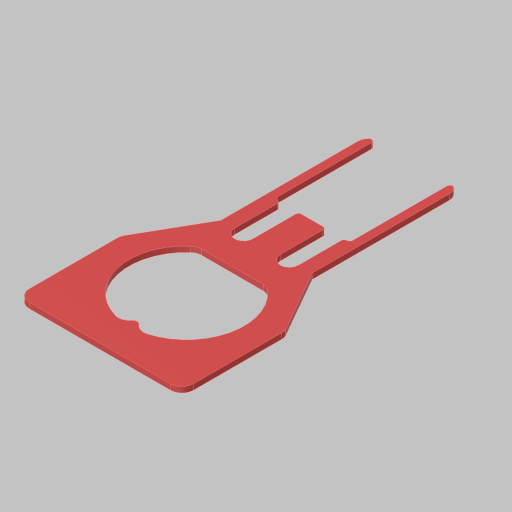
# Autodesk Inventor part: EL2-037
Saved by Autodesk Inventor 2023.5 (Build 275446000, 446)
## iProperties
Created: 2025-01-21
Part Number: EL2-037
Material: ABS Plastic
Document SubType Name: Modeling
Designer: slick
Density: 1.06 g/cm^3
Appearance: Smooth - Red
Author: slick
Autodesk Inventor part; units mm, degrees
ref_plane "YZ Plane" through (0, 0, 0) normal (1, 0, 0) x (0, 1, 0)
ref_plane "XZ Plane" through (0, 0, 0) normal (0, 1, 0) x (-1, 0, 0)
ref_plane "XY Plane" through (0, 0, 0) normal (0, 0, 1) x (1, 0, 0)
sketch "Sketch1" plane through (0, 0, 0) normal (0, 1, 0) x (-1, 0, 0)
  line L0 (8.89, 0) -> (-8.89, 0) construction
  line L1 (8.89, 1.5875) -> (-8.89, 1.5875)
  line L2 (-8.89, -1.5875) -> (8.89, -1.5875)
  arc A0 (8.89, -1.5875) -> (8.89, 1.5875) centre (8.89, 0) ccw
  arc A1 (-8.89, 1.5875) -> (-8.89, -1.5875) centre (-8.89, 0) ccw
  line L3 (8.89, -5.0038) -> (-8.89, -5.0038) construction
  line L4 (8.89, -3.4163) -> (-8.89, -3.4163)
  line L5 (-8.89, -6.5913) -> (8.89, -6.5913)
  arc A2 (8.89, -6.5913) -> (8.89, -3.4163) centre (8.89, -5.0038) ccw
  arc A3 (-8.89, -3.4163) -> (-8.89, -6.5913) centre (-8.89, -5.0038) ccw
  line L6 (8.89, -10.0076) -> (-8.89, -10.0076) construction
  line L7 (8.89, -8.4201) -> (-8.89, -8.4201)
  line L8 (-8.89, -11.5951) -> (8.89, -11.5951)
  arc A4 (8.89, -11.5951) -> (8.89, -8.4201) centre (8.89, -10.0076) ccw
  arc A5 (-8.89, -8.4201) -> (-8.89, -11.5951) centre (-8.89, -10.0076) ccw
  line L9 (12.7, 32.8549) -> (-12.7, 32.8549)
  line L10 (-12.7, 32.8549) -> (-12.7, -17.9451)
  line L11 (-12.7, -17.9451) -> (12.7, -17.9451)
  line L12 (12.7, -17.9451) -> (12.7, 32.8549)
  line L13 (6.35, 26.5049) -> (-6.35, 26.5049) construction
  arc A6 (8.89, -16.5989) -> (8.89, -13.4239) centre (8.89, -15.0114) ccw
  line L14 (-8.89, -16.5989) -> (8.89, -16.5989)
  arc A7 (-8.89, -13.4239) -> (-8.89, -16.5989) centre (-8.89, -15.0114) ccw
  line L15 (8.89, -13.4239) -> (-8.89, -13.4239)
  point P0 (0, 0)
  point P1 (0, -5.0038)
  point P2 (0, -10.0076)
  point P3 (10.4775, -5.0038)
  point P4 (10.4775, 0)
  point P5 (10.4775, -10.0076)
  point P6 (0, -17.9451)
  point P7 (0, -11.5951)
  point P8 (0, 26.5049)
  point P9 (0, 32.8549)
  point P10 (10.4775, -15.0114)
  point P11 (0, -16.5989)
  dimension "d1" = 17.78
  dimension "d3" = 3.175
  dimension "d4" = 5.0038
  dimension "d5" = 5.0038
  dimension "d8" = 25.4
  dimension "d9" = 50.8
  dimension "d10" = 6.35
  dimension "d11" = 12.7
  dimension "d12" = 6.35
  dimension "d43" = 5.0038
  constraints: 38 end point, 19 point on circle, 12 tangent, 9 parallel, 8 centre point, 7 midpoint, 4 vertical alignment, 3 horizontal, 2 equal radius, 1 horizontal alignment, 1 perpendicular, 1 vertical, 12 other
  measures "d1" distance of L1.start L1.end
  measures "d3" distance between parallel lines of L2 L1
  measures "d4" distance of point (10.477, -5.004) point (10.477, 0)
  measures "d5" distance of point (10.477, -10.008) point (10.477, -5.004)
  measures "d8" distance of L10.end L11.end
  measures "d9" distance of L11.end L9.start
  measures "d10" distance of point (0, -11.595) point (0, -17.945)
  measures "d11" distance of L13.start L13.end
  measures "d12" distance from line of L9 L13.start
  measures "d43" distance of L6.start A6.centre
extrude "Extrusion1" add sketch "Sketch1" along normal blind 6.35 contours A0 L2 A1 L1 | A2 L5 A3 L4 | A4 L8 A5 L7 | L12 L11 L10 L9 | L14 A7 L15 A6
fillet "Fillet1" radius 3.175 4 edges at (-12.7, 3.175, -17.9451) (12.7, 3.175, -17.9451) (12.7, 3.175, 32.8549) (-12.7, 3.175, 32.8549)
sketch "Sketch2" plane through (0, 6.35, 0) normal (0, 1, 0) x (1, 0, 0)
  line L0 (-6.35, -10.6299) -> (-6.35, -23.3299) construction
  line L1 (-8.9027, -10.6299) -> (-8.9027, -23.3299)
  line L2 (-3.7973, -23.3299) -> (-3.7973, -10.6299)
  arc A0 (-3.7973, -10.6299) -> (-8.9027, -10.6299) centre (-6.35, -10.6299) ccw
  arc A1 (-8.9027, -23.3299) -> (-3.7973, -23.3299) centre (-6.35, -23.3299) ccw
  line L3 (6.35, -10.6299) -> (6.35, -23.3299) construction
  line L4 (3.7973, -10.6299) -> (3.7973, -23.3299)
  line L5 (8.9027, -23.3299) -> (8.9027, -10.6299)
  arc A2 (8.9027, -10.6299) -> (3.7973, -10.6299) centre (6.35, -10.6299) ccw
  arc A3 (3.7973, -23.3299) -> (8.9027, -23.3299) centre (6.35, -23.3299) ccw
  line L6 (-9.525, -32.8549) -> (9.525, -32.8549) projected
  line L7 (9.525, 17.9451) -> (-9.525, 17.9451) projected
  line L8 (-6.35, -16.9799) -> (6.35, -16.9799) construction
  point P0 (0, 0)
  point P1 (0, -16.9799)
  point P2 (0, 17.9451)
  dimension "d23" = 5.1054
  dimension "d24" = 12.7
  dimension "d26" = 34.925
  dimension "d27" = 12.7
  constraints: 18 end point, 8 point on circle, 8 tangent, 4 centre point, 4 midpoint, 3 parallel, 2 horizontal alignment, 1 equal radius, 1 perpendicular, 1 vertical, 1 vertical alignment
  measures "d23" diameter of A1
  measures "d24" distance of L0.start L0.end
  measures "d26" distance from line of L8.start L7
  measures "d27" distance of L8.start L8.end
extrude "Extrusion2" cut sketch "Sketch2" against normal blind 25.4
sketch "Sketch3" plane through (0, 6.35, 0) normal (0, 1, 0) x (1, 0, 0)
  circle A0 centre (0, -45.5549) radius 16.002
  line L0 (-9.525, -32.8549) -> (9.525, -32.8549) projected
  circle A1 centre (0, -45.5549) radius 19.177
  line L1 (3.7973, -10.6299) -> (3.7973, -23.3299) projected
  arc A2 (3.7973, -23.3299) -> (8.9027, -23.3299) centre (6.35, -23.3299) ccw projected
  line L2 (8.9027, -23.3299) -> (8.9027, -10.6299) projected
  arc A3 (8.9027, -10.6299) -> (3.7973, -10.6299) centre (6.35, -10.6299) ccw projected
  line L3 (-8.9027, -10.6299) -> (-8.9027, -23.3299) projected
  arc A4 (-8.9027, -23.3299) -> (-3.7973, -23.3299) centre (-6.35, -23.3299) ccw projected
  line L4 (-3.7973, -23.3299) -> (-3.7973, -10.6299) projected
  arc A5 (-3.7973, -10.6299) -> (-8.9027, -10.6299) centre (-6.35, -10.6299) ccw projected
  arc A6 (-12.7, -29.6799) -> (-9.525, -32.8549) centre (-9.525, -29.6799) ccw projected
  line L5 (-12.7, -29.6799) -> (-12.7, 14.7701) projected
  arc A7 (-9.525, 17.9451) -> (-12.7, 14.7701) centre (-9.525, 14.7701) ccw projected
  line L6 (-9.525, 17.9451) -> (9.525, 17.9451) projected
  arc A8 (12.7, 14.7701) -> (9.525, 17.9451) centre (9.525, 14.7701) ccw projected
  line L7 (12.7, 14.7701) -> (12.7, -29.6799) projected
  arc A9 (9.525, -32.8549) -> (12.7, -29.6799) centre (9.525, -29.6799) ccw projected
  line L8 (9.525, -32.8549) -> (-9.525, -32.8549) projected
  line L9 (3.7973, -10.6299) -> (3.7973, -23.3299) projected
  arc A10 (3.7973, -23.3299) -> (8.9027, -23.3299) centre (6.35, -23.3299) ccw projected
  line L10 (8.9027, -23.3299) -> (8.9027, -10.6299) projected
  arc A11 (8.9027, -10.6299) -> (3.7973, -10.6299) centre (6.35, -10.6299) ccw projected
  line L11 (-8.9027, -10.6299) -> (-8.9027, -23.3299) projected
  arc A12 (-8.9027, -23.3299) -> (-3.7973, -23.3299) centre (-6.35, -23.3299) ccw projected
  line L12 (-3.7973, -23.3299) -> (-3.7973, -10.6299) projected
  arc A13 (-3.7973, -10.6299) -> (-8.9027, -10.6299) centre (-6.35, -10.6299) ccw projected
  arc A14 (-12.7, -29.6799) -> (-9.525, -32.8549) centre (-9.525, -29.6799) ccw projected
  line L13 (-12.7, -29.6799) -> (-12.7, 14.7701) projected
  arc A15 (-9.525, 17.9451) -> (-12.7, 14.7701) centre (-9.525, 14.7701) ccw projected
  line L14 (-9.525, 17.9451) -> (9.525, 17.9451) projected
  arc A16 (12.7, 14.7701) -> (9.525, 17.9451) centre (9.525, 14.7701) ccw projected
  line L15 (12.7, 14.7701) -> (12.7, -29.6799) projected
  arc A17 (9.525, -32.8549) -> (12.7, -29.6799) centre (9.525, -29.6799) ccw projected
  line L16 (9.525, -32.8549) -> (-9.525, -32.8549) projected
  point P0 (0, 0)
  point P1 (0, -32.8549)
  point P2 (12.433012, -30.954299)
  point P3 (9.726813, -32.84848)
  point P4 (-9.726813, -32.84848)
  point P5 (-12.433012, -30.954299)
  dimension "d30" = 32.004
  dimension "d31" = 12.7
  dimension "d32" = 3.175
  constraints: 2 centre point, 1 midpoint, 1 vertical alignment
  measures "d30" diameter of A0
  measures "d31" distance from line of L0 A0.centre
  measures "d32" radial gap between concentric circles of A0 A1
extrude "Extrusion3" add sketch "Sketch3" against normal up to surface (6.35 mm away) contours A0 A9 A1 A6 picked at (17.941917, -47.047698)
fillet "Fillet2" radius 3.175 4 edges at (-12.433, 3.175, 30.9543) (12.433, 3.175, 30.9543) (9.7268, 3.175, 32.8485) (-9.7268, 3.175, 32.8485)
sketch "Sketch4" plane through (0, 6.35, 0) normal (0, 1, 0) x (1, 0, 0)
  circle A0 centre (0, -60.4901) radius 1.1811
  arc A1 (-8.59106, -32.8549) -> (-10.717559, -33.672227) centre (-8.59106, -36.0299) ccw
  arc A2 (-10.717559, -33.672227) -> (10.717559, -33.672227) centre (0, -45.5549) ccw
  arc A3 (10.717559, -33.672227) -> (8.59106, -32.8549) centre (8.59106, -36.0299) ccw
  line L0 (8.59106, -32.8549) -> (-8.59106, -32.8549)
  arc A4 (12.699247, -29.749044) -> (13.618736, -32.053517) centre (15.873494, -29.818188) ccw
  arc A5 (-13.618736, -32.053517) -> (13.618736, -32.053517) centre (0, -45.5549) ccw
  arc A6 (-13.618736, -32.053517) -> (-12.699247, -29.749044) centre (-15.873494, -29.818188) ccw
  arc A7 (-12.7, -29.6799) -> (-12.699247, -29.749044) centre (-9.525, -29.6799) ccw
  line L1 (-12.7, -29.6799) -> (-12.7, 14.7701)
  arc A8 (-9.525, 17.9451) -> (-12.7, 14.7701) centre (-9.525, 14.7701) ccw
  line L2 (-9.525, 17.9451) -> (9.525, 17.9451)
  arc A9 (12.7, 14.7701) -> (9.525, 17.9451) centre (9.525, 14.7701) ccw
  line L3 (12.7, 14.7701) -> (12.7, -29.6799)
  arc A10 (12.699247, -29.749044) -> (12.7, -29.6799) centre (9.525, -29.6799) ccw
  line L4 (3.7973, -10.6299) -> (3.7973, -23.3299)
  arc A11 (3.7973, -23.3299) -> (8.9027, -23.3299) centre (6.35, -23.3299) ccw
  line L5 (8.9027, -23.3299) -> (8.9027, -10.6299)
  arc A12 (8.9027, -10.6299) -> (3.7973, -10.6299) centre (6.35, -10.6299) ccw
  line L6 (-8.9027, -10.6299) -> (-8.9027, -23.3299)
  arc A13 (-8.9027, -23.3299) -> (-3.7973, -23.3299) centre (-6.35, -23.3299) ccw
  line L7 (-3.7973, -23.3299) -> (-3.7973, -10.6299)
  arc A14 (-3.7973, -10.6299) -> (-8.9027, -10.6299) centre (-6.35, -10.6299) ccw
  point P0 (0, 0)
  point P1 (0, -61.5569)
  point P2 (-0.524608, -61.548298)
  point P3 (0.524608, -61.548298)
  dimension "d36" = 2.3622
  dimension "d37" = 1.0668
  constraints: 1 centre point, 1 point on circle
  measures "d36" diameter of A0
  measures "d37" distance of point (0, -61.557) A0.centre
extrude "Extrusion4" add sketch "Sketch4" against normal up to surface (6.35 mm away) contours A0 A2 picked at (-0.032567, -60.808312)
fillet "Fillet3" radius 3.175 2 edges at (0.5246, 3.175, 61.5483) (-0.5246, 3.175, 61.5483)
sketch "Sketch5" plane through (0, 6.35, 0) normal (0, 1, 0) x (1, 0, 0)
  arc A0 (-8.59106, -32.8549) -> (-10.717559, -33.672227) centre (-8.59106, -36.0299) ccw construction
  arc A1 (-10.717559, -33.672227) -> (-4.36514, -60.950015) centre (0, -45.5549) ccw construction
  arc A2 (-4.36514, -60.950015) -> (-0.94872, -59.786588) centre (-3.499041, -57.895428) ccw construction
  arc A3 (0.94872, -59.786588) -> (-0.94872, -59.786588) centre (0, -60.4901) ccw construction
  arc A4 (0.94872, -59.786588) -> (4.36514, -60.950015) centre (3.499041, -57.895428) ccw construction
  arc A5 (4.36514, -60.950015) -> (10.717559, -33.672227) centre (0, -45.5549) ccw construction
  arc A6 (10.717559, -33.672227) -> (8.59106, -32.8549) centre (8.59106, -36.0299) ccw construction
  line L0 (8.59106, -32.8549) -> (-8.59106, -32.8549) construction
  arc A7 (12.699247, -29.749044) -> (13.618736, -32.053517) centre (15.873494, -29.818188) ccw construction
  arc A8 (-13.618736, -32.053517) -> (13.618736, -32.053517) centre (0, -45.5549) ccw construction
  arc A9 (-13.618736, -32.053517) -> (-12.699247, -29.749044) centre (-15.873494, -29.818188) ccw construction
  arc A10 (-12.7, -29.6799) -> (-12.699247, -29.749044) centre (-9.525, -29.6799) ccw construction
  line L1 (-12.7, -29.6799) -> (-12.7, 14.7701) construction
  arc A11 (-9.525, 17.9451) -> (-12.7, 14.7701) centre (-9.525, 14.7701) ccw construction
  line L2 (-9.525, 17.9451) -> (9.525, 17.9451) construction
  arc A12 (12.7, 14.7701) -> (9.525, 17.9451) centre (9.525, 14.7701) ccw construction
  line L3 (12.7, 14.7701) -> (12.7, -29.6799) construction
  arc A13 (12.699247, -29.749044) -> (12.7, -29.6799) centre (9.525, -29.6799) ccw construction
  line L4 (3.7973, -10.6299) -> (3.7973, -23.3299) construction
  arc A14 (3.7973, -23.3299) -> (8.9027, -23.3299) centre (6.35, -23.3299) ccw construction
  line L5 (8.9027, -23.3299) -> (8.9027, -10.6299) construction
  arc A15 (8.9027, -10.6299) -> (3.7973, -10.6299) centre (6.35, -10.6299) ccw construction
  line L6 (-8.9027, -10.6299) -> (-8.9027, -23.3299) construction
  arc A16 (-8.9027, -23.3299) -> (-3.7973, -23.3299) centre (-6.35, -23.3299) ccw construction
  line L7 (-3.7973, -23.3299) -> (-3.7973, -10.6299) construction
  arc A17 (-3.7973, -10.6299) -> (-8.9027, -10.6299) centre (-6.35, -10.6299) ccw construction
  line L8 (-22.86, -21.4249) -> (22.86, -21.4249)
  line L9 (22.86, -21.4249) -> (22.86, -69.6849)
  line L10 (22.86, -69.6849) -> (-22.86, -69.6849)
  line L11 (-22.86, -69.6849) -> (-22.86, -21.4249)
  line L12 (-22.86, -21.4249) -> (22.86, -69.6849) construction
  line L13 (22.86, -21.4249) -> (-22.86, -69.6849) construction
  line L14 (-22.86, -41.1099) -> (-12.7, -23.3299)
  line L15 (-12.7, 14.7701) -> (-12.7, -29.6799) construction
  line L16 (12.7, -29.6799) -> (12.7, 14.7701) construction
  line L17 (12.7, -23.3299) -> (22.86, -41.1099)
  arc A18 (-13.618736, -32.053517) -> (-12.699247, -29.749044) centre (-15.873494, -29.818188) ccw construction
  arc A19 (-13.618736, -32.053517) -> (13.618736, -32.053517) centre (0, -45.5549) ccw construction
  arc A20 (-13.618736, -32.053517) -> (13.618736, -32.053517) centre (0, -45.5549) ccw
  arc A21 (12.699247, -29.749044) -> (13.618736, -32.053517) centre (15.873494, -29.818188) ccw
  arc A22 (-13.586812, -32.021391) -> (-12.699812, -29.714474) centre (-15.873494, -29.818188) ccw
  arc A23 (-12.7, -29.6799) -> (-12.699247, -29.749044) centre (-9.525, -29.6799) ccw construction
  line L18 (-13.586812, -32.021391) -> (-13.618736, -32.053517)
  line L19 (-12.7, -23.3299) -> (-12.699812, -29.714474)
  line L20 (12.7, -23.3299) -> (12.7, -29.6799)
  arc A24 (12.699247, -29.749044) -> (12.7, -29.6799) centre (9.525, -29.6799) ccw construction
  line L21 (12.7, -29.915967) -> (12.7, -29.6799)
  point P0 (0, 0)
  dimension "d48" = 45.72
  dimension "d49" = 87.63
  dimension "d50" = 28.575
  constraints: 24 end point, 9 point on circle, 4 point on line, 3 centre point, 3 coincident, 3 horizontal alignment, 2 midpoint, 2 parallel, 2 tangent, 1 collinear, 1 horizontal, 1 perpendicular, 1 vertical
  measures "d48" distance of L9.end L10.end
  measures "d49" distance between parallel lines of L10 L2
  measures "d50" distance of L9.end L17.end
sketch "Sketch5 outline for Extrusion5" plane through (0, 6.35, 0) normal (0, 1, 0) x (1, 0, 0)
  line L0 (-22.86, -69.6849) -> (22.86, -69.6849)
  line L1 (-22.86, -41.1099) -> (-22.86, -69.6849)
  line L2 (-12.7, -23.3299) -> (-22.86, -41.1099)
  line L3 (-12.699812, -29.714474) -> (-12.7, -23.3299)
  arc A0 (-13.586812, -32.021391) -> (-12.699812, -29.714474) centre (-15.873494, -29.818188) ccw
  line L4 (-13.618736, -32.053517) -> (-13.586812, -32.021391)
  arc A1 (13.618736, -32.053517) -> (-13.618736, -32.053517) centre (0, -45.5549) cw
  arc A2 (12.7, -29.915967) -> (13.618736, -32.053517) centre (15.873494, -29.818188) ccw
  line L5 (12.7, -29.6799) -> (12.7, -29.915967)
  line L6 (12.7, -23.3299) -> (12.7, -29.6799)
  line L7 (22.86, -41.1099) -> (12.7, -23.3299)
  line L8 (22.86, -69.6849) -> (22.86, -41.1099)
extrude "Extrusion5" add sketch "Sketch5 outline for Extrusion5" against normal up to surface (6.35 mm away)
fillet "Fillet4" radius 3.175 4 edges at (-22.86, 3.175, 41.1099) (22.86, 3.175, 41.1099) (22.86, 3.175, 69.6849) (-22.86, 3.175, 69.6849)
extrude "Extrusion7" cut sketch "Sketch1" along normal blind 4.318 contours A0 L2 A1 L1 | A2 L5 A3 L4 | A4 L8 A5 L7 | L14 A7 L15 A6
sketch "Sketch7" plane through (0, 0, 0) normal (0, -1, 0) x (1, 0, 0)
  line L0 (8.89, -3.4163) -> (-8.89, -3.4163) construction
  arc A0 (-8.89, -3.4163) -> (-8.89, -6.5913) centre (-8.89, -5.0038) ccw construction
  line L1 (-8.89, -6.5913) -> (8.89, -6.5913) construction
  arc A1 (8.89, -6.5913) -> (8.89, -3.4163) centre (8.89, -5.0038) ccw construction
  line L2 (8.89, -8.4201) -> (-8.89, -8.4201) construction
  arc A2 (-8.89, -8.4201) -> (-8.89, -11.5951) centre (-8.89, -10.0076) ccw construction
  line L3 (-8.89, -11.5951) -> (8.89, -11.5951) construction
  arc A3 (8.89, -11.5951) -> (8.89, -8.4201) centre (8.89, -10.0076) ccw construction
  line L4 (8.89, 1.5875) -> (-8.89, 1.5875) construction
  arc A4 (-8.89, 1.5875) -> (-8.89, -1.5875) centre (-8.89, 0) ccw construction
  line L5 (-8.89, -1.5875) -> (8.89, -1.5875) construction
  arc A5 (8.89, -1.5875) -> (8.89, 1.5875) centre (8.89, 0) ccw construction
  arc A6 (-8.89, -13.4239) -> (-8.89, -16.5989) centre (-8.89, -15.0114) ccw construction
  line L6 (-8.89, -16.5989) -> (8.89, -16.5989) construction
  arc A7 (8.89, -16.5989) -> (8.89, -13.4239) centre (8.89, -15.0114) ccw construction
  line L7 (8.89, -13.4239) -> (-8.89, -13.4239) construction
  arc A8 (22.86, 66.5099) -> (19.685, 69.6849) centre (19.685, 66.5099) ccw construction
  line L8 (22.86, 66.5099) -> (22.86, 41.953067) construction
  arc A9 (22.441672, 40.377826) -> (22.86, 41.953067) centre (19.685, 41.953067) ccw construction
  line L9 (22.441672, 40.377826) -> (12.7, 23.3299) construction
  line L10 (12.7, 23.3299) -> (12.7, -14.7701) construction
  arc A10 (9.525, -17.9451) -> (12.7, -14.7701) centre (9.525, -14.7701) ccw construction
  line L11 (9.525, -17.9451) -> (-9.525, -17.9451) construction
  arc A11 (-12.7, -14.7701) -> (-9.525, -17.9451) centre (-9.525, -14.7701) ccw construction
  line L12 (-12.7, -14.7701) -> (-12.7, 23.3299) construction
  line L13 (-12.7, 23.3299) -> (-22.441672, 40.377826) construction
  arc A12 (-22.86, 41.953067) -> (-22.441672, 40.377826) centre (-19.685, 41.953067) ccw construction
  line L14 (-22.86, 41.953067) -> (-22.86, 66.5099) construction
  arc A13 (-19.685, 69.6849) -> (-22.86, 66.5099) centre (-19.685, 66.5099) ccw construction
  line L15 (-19.685, 69.6849) -> (19.685, 69.6849) construction
  line L16 (12.7, 29.6799) -> (12.7, 29.915967) construction
  arc A14 (12.7, 29.915967) -> (12.699247, 29.749044) centre (15.873494, 29.818188) ccw construction
  arc A15 (12.7, 29.6799) -> (12.699247, 29.749044) centre (9.525, 29.6799) ccw construction
  arc A16 (-10.717559, 33.672227) -> (-8.59106, 32.8549) centre (-8.59106, 36.0299) ccw construction
  line L17 (-8.59106, 32.8549) -> (8.59106, 32.8549) construction
  arc A17 (8.59106, 32.8549) -> (10.717559, 33.672227) centre (8.59106, 36.0299) ccw construction
  arc A18 (10.717559, 33.672227) -> (4.36514, 60.950015) centre (0, 45.5549) ccw construction
  arc A19 (4.36514, 60.950015) -> (0.94872, 59.786588) centre (3.499041, 57.895428) ccw construction
  arc A20 (-0.94872, 59.786588) -> (0.94872, 59.786588) centre (0, 60.4901) ccw construction
  arc A21 (-0.94872, 59.786588) -> (-4.36514, 60.950015) centre (-3.499041, 57.895428) ccw construction
  arc A22 (-4.36514, 60.950015) -> (-10.717559, 33.672227) centre (0, 45.5549) ccw construction
  line L18 (3.7973, 23.3299) -> (3.7973, 10.6299) construction
  arc A23 (3.7973, 10.6299) -> (8.9027, 10.6299) centre (6.35, 10.6299) ccw construction
  line L19 (8.9027, 10.6299) -> (8.9027, 23.3299) construction
  arc A24 (8.9027, 23.3299) -> (3.7973, 23.3299) centre (6.35, 23.3299) ccw construction
  line L20 (-8.9027, 23.3299) -> (-8.9027, 10.6299) construction
  arc A25 (-8.9027, 10.6299) -> (-3.7973, 10.6299) centre (-6.35, 10.6299) ccw construction
  line L21 (-3.7973, 10.6299) -> (-3.7973, 23.3299) construction
  arc A26 (-3.7973, 23.3299) -> (-8.9027, 23.3299) centre (-6.35, 23.3299) ccw construction
  line L22 (10.4775, -17.9451) -> (-10.4775, -17.9451)
  line L23 (-10.4775, -17.9451) -> (-10.4775, 10.6299)
  line L24 (-10.4775, 10.6299) -> (10.4775, 10.6299)
  line L25 (10.4775, 10.6299) -> (10.4775, -17.9451)
  arc A27 (8.89, -16.5989) -> (8.89, -13.4239) centre (8.89, -15.0114) ccw construction
  line L26 (9.525, -17.9451) -> (-9.525, -17.9451) construction
  point P0 (0, 0)
  point P1 (10.4775, -15.0114)
  point P2 (-10.4775, -15.0114)
  point P3 (0, -17.9451)
  point P4 (0, 10.6299)
  constraints: 8 end point, 3 midpoint, 2 parallel, 2 point on circle, 2 point on line, 1 horizontal, 1 horizontal alignment, 1 perpendicular
extrude "Extrusion8" cut sketch "Sketch7" against normal blind 1.524
fillet "Fillet5" radius 0.79375 8 edges at (10.4775, 0.762, -17.7989) (-10.4775, 0.762, -17.7989) (-10.4775, 0.762, 10.6299) (10.4775, 0.762, 10.6299) (8.9027, 0.762, 10.6299) (3.7973, 0.762, 10.6299) (-3.7973, 0.762, 10.6299) (-8.9027, 0.762, 10.6299)
sketch "Sketch8" plane through (0, 6.35, 0) normal (0, 1, 0) x (1, 0, 0)
  line L0 (-108.579941, 52.506068) -> (91.97877, 52.506068)
  line L1 (91.97877, 52.506068) -> (91.97877, -83.146187)
  line L2 (91.97877, -83.146187) -> (-108.579941, -83.146187)
  line L3 (-108.579941, -83.146187) -> (-108.579941, 52.506068)
  point P0 (0, 0)
  constraints: 8 end point, 2 parallel, 1 horizontal, 1 perpendicular
extrude "Extrusion9" cut sketch "Sketch8" against normal up to surface (4.826 mm away)
equation "\"d5\" = d4"
equation "\"d43\" = d5"
body "Solid1"
